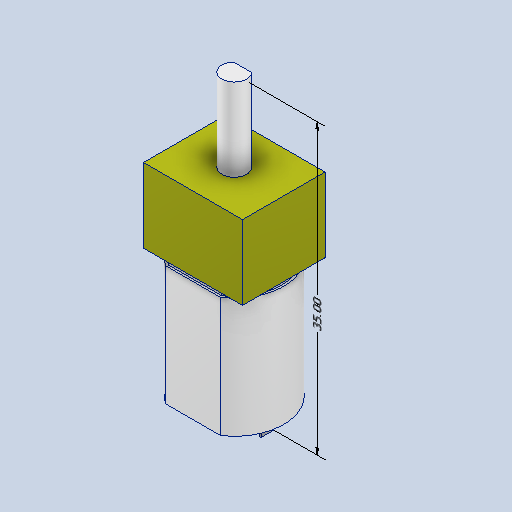
# Autodesk Inventor part: motor_6V_60RPM
Saved by Autodesk Inventor 2024.1 (Build 281209000, 209)
## iProperties
Created: 2025-01-16
Part Number: motor_6V_60RPM
Material: アルミニウム 6061
Document SubType Name: Modeling
Designer: hibik
Density: 2.7 g/cm^3
Appearance: アルミニウム - フラット
Author: hibik
Autodesk Inventor part; units mm, degrees
ref_plane "YZ Plane" through (0, 0, 0) normal (1, 0, 0) x (0, 1, 0)
ref_plane "XZ Plane" through (0, 0, 0) normal (0, 1, 0) x (-1, 0, 0)
ref_plane "XY Plane" through (0, 0, 0) normal (0, 0, 1) x (1, 0, 0)
sketch "スケッチ1" plane through (0, 0, 0) normal (0, 1, 0) x (-1, 0, 0)
  circle A0 centre (0, 0) radius 6
  line L0 (3.3166, 5) -> (-3.3166, 5)
  line L1 (-3.3166, 5) -> (-3.3166, -5)
  line L2 (-3.3166, -5) -> (3.3166, -5)
  line L3 (3.3166, -5) -> (3.3166, 5)
  dimension "d0" = 12
  dimension "d1" = 10
  constraints: 8 end point, 3 point on circle, 2 parallel, 1 centre point, 1 coincident, 1 horizontal, 1 perpendicular
  measures "d0" diameter of A0
  measures "d1" distance of L2.end L0.start
extrude "押し出し1" add sketch "スケッチ1" along normal blind 15 contours A0 L3 | L3 L2 L1 L0 | L1 A0
sketch "スケッチ2" plane through (0, 0, 0) normal (0, -1, 0) x (1, 0, 0)
  circle A0 centre (0, 0) radius 2.5
  dimension "d4" = 5
  constraints: 1 centre point, 1 coincident
  measures "d4" diameter of A0
extrude "押し出し2" add sketch "スケッチ2" along normal blind 1
sketch "スケッチ3" plane through (0, 0, 0) normal (0, -1, 0) x (1, 0, 0)
  line L0 (4, -0.75) -> (-4, -0.75)
  line L1 (-4, -0.75) -> (-4, 0.75)
  line L2 (-4, 0.75) -> (4, 0.75)
  line L3 (4, 0.75) -> (4, -0.75)
  line L4 (3.75, -0.75) -> (-3.75, -0.75)
  line L5 (-3.75, -0.75) -> (-3.75, 0.75)
  line L6 (-3.75, 0.75) -> (3.75, 0.75)
  line L7 (3.75, 0.75) -> (3.75, -0.75)
  point P0 (0, 0)
  point P1 (4, 0)
  point P2 (0, -0.75)
  point P3 (0, 0.75)
  dimension "d7" = 8
  dimension "d8" = 1.5
  dimension "d9" = 7.5
  constraints: 16 end point, 4 midpoint, 4 parallel, 2 horizontal, 2 perpendicular, 2 point on line, 1 horizontal alignment, 1 vertical alignment
  measures "d7" distance of L1.end L2.end
  measures "d8" distance of L0.end L1.end
  measures "d9" distance of L5.end L6.end
extrude "押し出し3" add sketch "スケッチ3" along normal blind 2 contours L0 L7 L2 L3 | L0 L1 L2 L5
sketch "スケッチ4" plane through (0, 15, 0) normal (0, 1, 0) x (1, 0, 0)
  line L0 (-6, 5) -> (6, 5)
  line L1 (6, 5) -> (6, -5)
  line L2 (6, -5) -> (-6, -5)
  line L3 (-6, -5) -> (-6, 5)
  line L4 (3.3166, 5) -> (-3.3166, 5) projected
  arc A0 (3.3166, -5) -> (3.3166, 5) centre (0, 0) ccw projected
  arc A1 (-3.3166, 5) -> (-3.3166, -5) centre (0, 0) ccw projected
  line L5 (-3.3166, -5) -> (3.3166, -5) projected
  constraints: 8 end point, 2 collinear, 2 parallel, 2 tangent, 1 horizontal, 1 perpendicular
extrude "押し出し4" add sketch "スケッチ4" along normal blind 9
sketch "スケッチ5" plane through (0, 24, 0) normal (0, 1, 0) x (1, 0, 0)
  circle A0 centre (0, 0) radius 1.5
  line L0 (-1.118, 1) -> (1.118, 1)
  dimension "d14" = 3
  dimension "d27" = 1
  constraints: 2 end point, 2 point on circle, 1 centre point, 1 coincident, 1 horizontal
  measures "d14" diameter of A0
  measures "d27" distance from line of point (0, 0) L0
extrude "押し出し5" add sketch "スケッチ5" along normal blind 10 contours A0 L0 picked at (0.0594, 0.1702)
sketch "スケッチ6" plane through (0, 15, 0) normal (0, -1, 0) x (1, 0, 0)
  arc A0 (6, 0) -> (3.3166, 5) centre (0, 0) ccw projected
  line L0 (6, 5) -> (6, 0) projected
  line L1 (3.3166, 5) -> (6, 5) projected
  arc A1 (3.3166, -5) -> (6, 0) centre (0, 0) ccw projected
  line L2 (6, -5) -> (3.3166, -5) projected
  line L3 (6, 0) -> (6, -5) projected
  arc A2 (-6, 0) -> (-3.3166, -5) centre (0, 0) ccw projected
  line L4 (-6, -5) -> (-6, 0) projected
  line L5 (-3.3166, -5) -> (-6, -5) projected
  arc A3 (-3.3166, 5) -> (-6, 0) centre (0, 0) ccw projected
  line L6 (-6, 5) -> (-3.3166, 5) projected
  line L7 (-6, 0) -> (-6, 5) projected
  arc A4 (1.118, -1) -> (-1.118, -1) centre (0, 0) ccw projected
  line L8 (-6, -5) -> (-6, 5) projected
  line L9 (-6, 5) -> (6, 5) projected
  line L10 (6, 5) -> (6, -5) projected
  line L11 (6, -5) -> (-6, -5) projected
  circle A5 centre (0, 0) radius 5.75
  line L12 (3.2404, -4.75) -> (-3.2404, -4.75)
  line L13 (-3.2404, -4.75) -> (-3.2404, 4.75)
  line L14 (-3.2404, 4.75) -> (3.2404, 4.75)
  line L15 (3.2404, 4.75) -> (3.2404, -4.75)
  line L16 (-1.118, -1) -> (1.118, -1) projected
  point P0 (-3.3166, -5)
  point P1 (3.3166, -5)
  dimension "d17" = 11.5
  dimension "d18" = 9.5
  constraints: 8 end point, 3 point on circle, 2 parallel, 1 centre point, 1 coincident, 1 horizontal, 1 perpendicular
  measures "d17" diameter of A5
  measures "d18" distance between parallel lines of L14 L12
extrude "押し出し6" cut sketch "スケッチ6" along normal blind 0.5 contours A1 L11 A5 L9 A0 | A0 L1 L0 | L3 L2 A1 | A5 L14 L9 | L11 A5 L12 | A5 L11 A2 A3 L9 | A3 L7 L6 | L5 L4 A2
